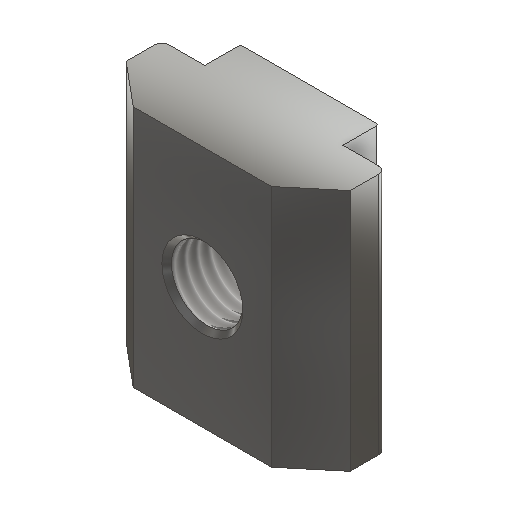
# Autodesk Inventor part: COTS_GENERIC_20x20_M3_Nut
Saved by Autodesk Inventor 2026.1 (Build 301233000, 233)
## iProperties
Created: 2016-10-26
Part Number: COTS_GENERIC_20x20_M3_Nut
Material: Сталь
Document SubType Name: Modeling
Designer: skhalipa
Density: 7.85 g/cm^3
Appearance: Сталь — полированная
Author: skhalipa
Autodesk Inventor part; units mm, degrees
ref_plane "YZ Plane" through (0, 0, 0) normal (1, 0, 0) x (0, 1, 0)
ref_plane "XZ Plane" through (0, 0, 0) normal (0, 1, 0) x (-1, 0, 0)
ref_plane "XY Plane" through (0, 0, 0) normal (0, 0, 1) x (1, 0, 0)
sketch "Эскиз1" plane through (0, 0, 0) normal (0, 0, 1) x (1, 0, 0)
  line L0 (-4.7, 2.25) -> (4.7, 2.25)
  line L1 (4.7, 2.25) -> (4.7, -2.25)
  line L2 (4.7, -2.25) -> (-4.7, -2.25)
  line L3 (-4.7, -2.25) -> (-4.7, 2.25)
  point P0 (0, 0)
  point P1 (-4.7, 0)
  point P2 (0, 2.25)
  dimension "d0" = 9.4
  dimension "d1" = 4.5
  constraints: 8 end point, 2 midpoint, 2 parallel, 1 horizontal, 1 horizontal alignment, 1 perpendicular, 1 vertical alignment
  measures "d0" distance of L0.start L0.end
  measures "d1" distance of L2.end L0.start
extrude "Выдавливание1" add sketch "Эскиз1" along normal mid plane 10.2
sketch "Эскиз3" plane through (0, 0, 5.1) normal (0, 0, 1) x (1, 0, 0)
  line L0 (-4.7, 2.25) -> (-4.7, -2.25) projected
  line L1 (-4.7, 0.75) -> (-2.9, 0.75)
  line L2 (-2.9, 0.75) -> (-2.9, 2.25)
  line L3 (4.7, 2.25) -> (-4.7, 2.25) projected
  line L4 (4.7, -2.25) -> (4.7, 2.25) projected
  line L5 (4.7, 0.75) -> (2.9, 0.75)
  line L6 (2.9, 0.75) -> (2.9, 2.25)
  point P0 (0, 0)
  dimension "d7" = 1.5
  dimension "d8" = 2.9
  dimension "d9" = 5.8
  constraints: 8 end point, 4 point on line, 2 horizontal, 2 perpendicular, 1 horizontal alignment
  measures "d7" distance of L5.end L6.end
  measures "d8" distance from line of point (0, 0) L2
  measures "d9" distance between parallel lines of L6 L2
extrude "Выдавливание2" cut sketch "Эскиз3" against normal blind 10.2
sketch "Эскиз5" plane through (0, 0, 5.1) normal (0, 0, 1) x (1, 0, 0)
  line L0 (-4.7, -2.25) -> (4.7, -2.25) projected
  line L1 (-2.9, -2.25) -> (-4.7, -0.75)
  line L2 (-4.7, 0.75) -> (-4.7, -2.25) projected
  line L3 (4.7, -2.25) -> (4.7, 0.75) projected
  line L4 (4.7, -0.75) -> (2.9, -2.25)
  point P0 (0, 0)
  dimension "d15" = 1.5
  dimension "d16" = 2.9
  dimension "d17" = 5.8
  constraints: 4 end point, 2 horizontal alignment, 2 midpoint, 2 point on line
  measures "d15" distance from line of L0 L1.end
  measures "d16" horizontal distance of point (0, 0) L1.start
  measures "d17" distance of L4.end L1.start
extrude "Выдавливание3" cut sketch "Эскиз5" against normal blind 10.2
sketch "Эскиз6" plane through (-2.9, 2.25, -5.1) normal (0, 1, 0) x (1, 0, 0)
  point P0 (2.9, -5.1)
  point P1 (2.9, -5.1)
  constraints: 1 coincident
hole "Отверстие1" at (0, 2.25, 0) direction (0, -1, 0) diameter 3 end through all
thread "Резьба1" size "M3x0.5" class "6H" standard "ANSI Metric M Profile" full length
chamfer "Фаска1" distance 0.2 angle 45 2 edges at (0, 2.25, -1.5) (0, -2.25, -1.5)
fillet "Сопряжение2" radius 0.1 2 edges at (2.9, 2.25, 0) (-2.9, 2.25, 0)
fillet "Сопряжение3" radius 0.3 2 edges at (-4.7, 0.75, 0) (4.7, 0.75, 0)
